Autodesk Inventor part; units mm, degrees
(part 2 of 2)
sketch "Sketch63" plane through (1746.7139, 341.0183, -3045.3822) normal (0, 1, 0) x (-1, 0, 0)
  line L0 (2814.4647, 31.5167) -> (3537.2629, -710.2842) projected
  line L1 (2814.4647, 31.5167) -> (3564.3033, -738.0355)
  line L2 (3564.3033, -738.0355) -> (3573.4709, -729.1027)
  line L3 (3573.4709, -729.1027) -> (2823.6324, 40.4494)
  line L4 (2823.6324, 40.4494) -> (2814.4647, 31.5167)
  point P0 (1746.7139, 3045.3822)
  dimension "d209" = 12.8
  constraints: 8 end point, 2 perpendicular, 1 collinear, 1 parallel
  measures "d209" distance between parallel lines of L3 L1
revolve "Revolution18" add sketch "Sketch63" angle 360 about axis through (-1826.757, 341.0183, -3774.4849) along (0.6978736, 0, 0.716221) separate body
sketch "Sketch64" plane through (0, 0, 0) normal (0, 0, 1) x (1, 0, 0)
  line L0 (196.7139, 1222.2183) -> (1196.7139, 1222.2183)
  line L1 (1196.7139, 1222.2183) -> (1196.7139, -867.7817)
  line L2 (1196.7139, -867.7817) -> (196.7139, -867.7817)
  line L3 (196.7139, -867.7817) -> (196.7139, 1222.2183)
  line L4 (-3223.2861, 2012.2183) -> (3796.7139, 2012.2183) projected
  line L5 (-3223.2861, -1587.7817) -> (-3223.2861, 2012.2183) projected
  point P0 (0, 0)
  dimension "d211" = 790
  dimension "d212" = 2090
  dimension "d213" = 1000
  dimension "d214" = 3420
  constraints: 8 end point, 2 parallel, 1 horizontal, 1 perpendicular
  measures "d211" distance between parallel lines of L0 L4
  measures "d212" distance between parallel lines of L2 L0
  measures "d213" distance between parallel lines of L1 L3
  measures "d214" distance between parallel lines of L5 L3
ref_plane "Work Plane39" through (1196.7139, 1222.2183, 0) normal (1, 0, 0) x (0, 1, 0)
sketch "Sketch65" plane through (1196.7139, 1222.2183, 0) normal (1, 0, 0) x (0, 1, 0)
  line L0 (0, 0) -> (-2090, 0) projected
  line L1 (0, 0) -> (-2090, 0)
  line L2 (-2090, 0) -> (-2090, -100)
  line L3 (0, 0) -> (0, -100)
  line L4 (0, -100) -> (-2090, -100)
  point P0 (-1222.2183, 0)
  dimension "d215" = 100
  constraints: 8 end point, 3 equal length, 1 perpendicular
  measures "d215" distance between parallel lines of L0 L4
extrude "Extrusion19" add sketch "Sketch65" against normal blind 25 separate body
extrude "Extrusion20" add sketch "Sketch64" against normal blind 25 bodies 6
ref_plane "Work Plane40" through (196.7139, 1222.2183, -12.5) normal (1, 0, 0) x (0, 1, 0)
sketch "Sketch66" plane through (196.7139, 1222.2183, -12.5) normal (1, 0, 0) x (0, 1, 0)
  line L0 (0, 12.5) -> (-2090, 12.5) projected
  line L1 (-2090, 12.5) -> (-2090, -87.5) projected
  line L2 (-2090, -87.5) -> (0, -87.5) projected
  line L3 (0, -87.5) -> (0, 12.5) projected
  line L4 (0, 12.5) -> (0, -87.5)
  line L5 (-2090, -87.5) -> (0, -87.5)
  line L6 (-2090, -87.5) -> (-2090, 12.5)
  line L7 (0, 12.5) -> (-2090, 12.5)
  point P0 (-1222.2183, 12.5)
  point P1 (0, 12.5)
  point P2 (-2090, 12.5)
  constraints: 8 end point, 2 equal length, 2 perpendicular
extrude "Extrusion21" add sketch "Sketch66" along normal blind 25 separate body
ref_plane "Work Plane41" through (1196.7139, 1222.2183, -12.5) normal (0, 1, 0) x (-1, 0, 0)
sketch "Sketch67" plane through (1196.7139, 1222.2183, -12.5) normal (0, 1, 0) x (-1, 0, 0)
  line L0 (0, 12.5) -> (1000, 12.5) projected
  line L1 (1000, -87.5) -> (1000, 12.5) projected
  line L2 (0, -87.5) -> (0, 12.5) projected
  line L3 (1000, 12.5) -> (0, 12.5)
  line L4 (0, 12.5) -> (0, -87.5)
  line L5 (0, -87.5) -> (1000, -87.5)
  line L6 (1000, -87.5) -> (1000, 12.5)
  point P0 (1196.7139, 12.5)
  constraints: 8 end point, 3 perpendicular, 1 collinear
extrude "Extrusion22" add sketch "Sketch67" against normal blind 25 separate body
ref_plane "Work Plane42" through (221.7139, -867.7817, -100) normal (0, 1, 0) x (-1, 0, 0)
sketch "Sketch68" plane through (221.7139, -867.7817, -100) normal (0, 1, 0) x (-1, 0, 0)
  line L0 (0, 0) -> (0, 100) projected
  line L1 (-975, 100) -> (-975, 0) projected
  line L2 (25, 100) -> (-975, 100) projected
  line L3 (0, 100) -> (-975, 100)
  line L4 (-975, 100) -> (-975, 0)
  line L5 (-975, 0) -> (0, 0)
  line L6 (0, 0) -> (-22.4858, 100)
  point P0 (221.7139, 100)
  constraints: 8 end point, 2 perpendicular, 1 collinear, 1 point on line
extrude "Extrusion23" add sketch "Sketch68" along normal blind 25 separate body
sketch "Sketch69" plane through (0, 0, 0) normal (0, 0, -1) x (-1, 0, 0)
  line L0 (-3796.7139, 2012.2183) -> (-3796.7139, -1587.7817) projected
  line L1 (-3796.7139, -1587.7817) -> (3223.2861, -1587.7817) projected
  line L2 (-1226.7139, -342.7817) -> (-1396.7139, -342.7817)
  line L3 (-1396.7139, -342.7817) -> (-1396.7139, -647.7817)
  line L4 (-1396.7139, -647.7817) -> (-1226.7139, -647.7817)
  line L5 (-1226.7139, -647.7817) -> (-1226.7139, -342.7817)
  point P0 (0, 0)
  dimension "d226" = 2400
  dimension "d227" = 170
  dimension "d228" = 940
  dimension "d229" = 1245
  constraints: 8 end point, 2 parallel, 1 horizontal, 1 perpendicular
  measures "d226" distance between parallel lines of L0 L3
  measures "d227" distance between parallel lines of L5 L3
  measures "d228" distance between parallel lines of L1 L4
  measures "d229" distance between parallel lines of L1 L2
extrude "Extrusion24" add sketch "Sketch69" along normal blind 140 bodies 6
ref_plane "Work Plane43" through (1396.7139, -647.7817, -140) normal (0, 0, 1) x (1, 0, 0)
sketch "Sketch70" plane through (1396.7139, -647.7817, -140) normal (0, 0, 1) x (1, 0, 0)
  line L0 (0, 0) -> (0, 305) projected
  line L1 (-170, 0) -> (0, 0) projected
  line L2 (-170, 305) -> (-170, 0) projected
  line L3 (0, 305) -> (-170, 305) projected
  line L4 (0, 0) -> (-170, 0)
  line L5 (-170, 150) -> (0, 150)
  line L6 (0, 150) -> (0, 0)
  line L7 (-170, 150) -> (-170, 0)
  point P0 (-1396.7139, 647.7817)
  dimension "d232" = 150
  constraints: 8 end point, 3 equal length, 2 point on line, 1 perpendicular
  measures "d232" distance between parallel lines of L1 L5
extrude "Extrusion25" add sketch "Sketch70" against normal blind 3010 contours L1 L2 L5 L0 bodies 6
ref_plane "Work Plane44" through (1396.7139, -342.7817, -140) normal (-1, 0, 0) x (0, -1, 0)
sketch "Sketch71" plane through (1396.7139, -342.7817, -140) normal (-1, 0, 0) x (0, -1, 0)
  line L0 (155, 0) -> (0, 0) projected
  line L1 (155, 0) -> (155, -3010) projected
  line L2 (0, 0) -> (155, -165)
  line L3 (155, -196.0399) -> (155, 0)
  line L4 (155, 0) -> (0, 0)
  line L5 (305, 140) -> (0, 140) projected
  point P0 (-342.7817, 140)
  dimension "d235" = 305
  constraints: 6 end point, 2 point on line, 1 collinear, 1 perpendicular
  measures "d235" distance from line of L5 L2.end
extrude "Extrusion26" add sketch "Sketch71" along normal up to surface (170 mm away) bodies 6
body "Solid1"
body "Solid2"
body "Solid3"
body "Solid4"
body "Solid5"
body "Solid6"
body "Solid7"
body "Solid8"
body "Solid9"
body "Solid11"
body "Solid12"
body "Solid13"
body "Solid16"
body "Solid17"
body "Solid18"
body "Solid19"
body "Solid20"
body "Solid21"
body "Solid22"
body "Solid23"
body "Solid24"
body "Solid25"
body "Solid26"
body "Solid27"
body "Solid28"
body "Solid29"
body "Solid30"
body "Solid31"
body "Solid32"
body "Solid33"
body "Solid34"
body "Solid35"
body "Solid36"
body "Solid37"
body "Solid38"
body "Solid39"
body "Solid40"
body "Solid41"
